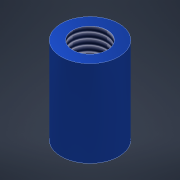
# Autodesk Inventor part: coupler
Saved by Autodesk Inventor 2021 (Build 250183000, 183)
## iProperties
Created: 2020-12-24
Part Number: coupler
Material: Generic
Document SubType Name: Modeling
Designer: Vikki
Density: 1 g/cm^3
Appearance: Anodized - Blue
Author: Vikki
Autodesk Inventor part; units mm, degrees
ref_plane "XZ Plane" through (0, 0, 0) normal (0, 1, 0) x (-1, 0, 0)
ref_plane "XY Plane" through (0, 0, 0) normal (0, 0, 1) x (1, 0, 0)
sketch "Sketch1" plane through (0, 0, 0) normal (0, 1, 0) x (-1, 0, 0)
  circle A0 centre (0, 0) radius 5
  dimension "d0" = 10
  constraints: 1 centre point, 1 coincident
  measures "d0" diameter of A0
extrude "Extrusion1" add sketch "Sketch1" along normal blind 18
sketch "Sketch2" plane through (0, 18, 0) normal (0, 1, 0) x (1, 0, 0)
  circle A0 centre (0, 0) radius 4
  circle A1 centre (0, 0) radius 5 projected
  dimension "d3" = 8
  constraints: 1 centre point, 1 coincident
  measures "d3" diameter of A0
extrude "Extrusion2" cut sketch "Sketch2" against normal blind 3
sketch "Sketch3" plane through (0, 18, 0) normal (0, 1, 0) x (1, 0, 0)
  circle A0 centre (0, 0) radius 3
  dimension "d6" = 6
  constraints: 1 centre point, 1 coincident
  measures "d6" diameter of A0
extrude "Extrusion3" cut sketch "Sketch3" against normal blind 12
sketch "Sketch4" plane through (0, 0, 0) normal (0, -1, 0) x (1, 0, 0)
  circle A0 centre (0, 0) radius 1.6
  dimension "d9" = 3.2
  constraints: 1 centre point, 1 coincident
  measures "d9" diameter of A0
extrude "Extrusion4" cut sketch "Sketch4" against normal blind 10
ref_plane "Work Plane1" through (-5, 0, 0) normal (1, 0, 0) x (0, 1, 0)
sketch "Sketch5" plane through (-5, 0, 0) normal (1, 0, 0) x (0, 1, 0)
  circle A0 centre (4, 0) radius 1.5
  line L0 (15, 5) -> (15, -5) projected
  point P0 (0, 0)
  dimension "d13" = 3
  dimension "d14" = 4
  constraints: 1 centre point, 1 horizontal alignment
  measures "d13" diameter of A0
  measures "d14" distance of point (0, 0) A0.centre
extrude "Extrusion5" cut sketch "Sketch5" along normal blind 5
sketch "Sketch6" plane through (0, 18, 0) normal (0, 1, 0) x (1, 0, 0)
  circle A0 centre (0, 0) radius 4 projected
extrude "Extrusion6" cut sketch "Sketch6" against normal up to surface (3 mm away)
thread "Thread1" size "M6x1" class "6H" standard "ANSI Metric M Profile" full length
body "Solid1"
